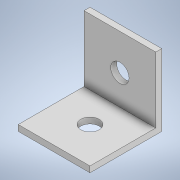
# Autodesk Inventor part: l-bracket
Saved by Autodesk Inventor 2020.1 (Build 241239000, 239)
## iProperties
Created: 2019-11-07
Part Number: l-bracket
Material: Generic
Document SubType Name: Modeling
Designer: amirs
Density: 1 g/cm^3
Appearance: Default
Author: amirs
Autodesk Inventor part; units mm, degrees
ref_plane "YZ Plane" through (0, 0, 0) normal (1, 0, 0) x (0, 1, 0)
ref_plane "XZ Plane" through (0, 0, 0) normal (0, 1, 0) x (-1, 0, 0)
ref_plane "XY Plane" through (0, 0, 0) normal (0, 0, 1) x (1, 0, 0)
sketch "Sketch1" plane through (0, 0, 0) normal (1, 0, 0) x (0, 1, 0)
  line L0 (0, 0) -> (0, 19.05)
  line L1 (0, 0) -> (19.05, 0)
  line L2 (1.5875, 19.05) -> (1.5875, 1.5875)
  line L3 (1.5875, 1.5875) -> (19.05, 1.5875)
  line L4 (0, 19.05) -> (1.5875, 19.05)
  line L5 (19.05, 0) -> (19.05, 1.5875)
  dimension "d0" = 19.05
  dimension "d1" = 19.05
  dimension "d2" = 1.5875
  constraints: 12 end point, 2 horizontal, 1 perpendicular, 1 vertical, 1 other
  measures "d0" distance of L0.start L1.end
  measures "d1" distance of L0.start L0.end
  measures "d2" distance between parallel lines of L0 L2
extrude "Extrusion1" add sketch "Sketch1" along normal blind 19.05
sketch "Sketch2" plane through (0, 0, 0) normal (0, -1, 0) x (1, 0, 0)
  line L0 (19.05, 1.5875) -> (19.05, 19.05) construction
  line L1 (19.05, 19.05) -> (0, 0) construction
  line L2 (0, 1.5875) -> (0, 19.05) construction
  line L3 (19.05, 0) -> (19.05, 1.5875) construction
  line L4 (0, 19.05) -> (19.05, 0) construction
  circle A0 centre (9.525, 9.525) radius 2.4384
  dimension "d5" = 4.8768
  constraints: 4 end point, 1 centre point, 1 midpoint
  measures "d5" diameter of A0
extrude "Extrusion2" cut sketch "Sketch2" against normal blind 25.4
sketch "Sketch3" plane through (0, 0, 0) normal (0, 0, -1) x (-1, 0, 0)
  line L0 (-19.05, 0) -> (-19.05, 19.05) construction
  line L1 (-19.05, 19.05) -> (0, 0) construction
  line L2 (0, 0) -> (0, 19.05) construction
  line L3 (0, 0) -> (-19.05, 0) construction
  line L4 (0, 19.05) -> (-19.05, 0) construction
  circle A0 centre (-9.525, 9.525) radius 2.4384
  dimension "d8" = 4.8768
  constraints: 4 end point, 1 centre point, 1 midpoint, 1 perpendicular
  measures "d8" diameter of A0
extrude "Extrusion3" cut sketch "Sketch3" against normal blind 25.4
body "Solid1"
